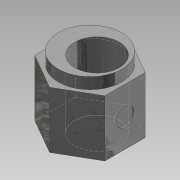
# Autodesk Inventor part: Eccentric M5 Spacer
Saved by Autodesk Inventor 2016 (Build 200138000, 138)
## iProperties
Created: 2013-06-19
Part Number: Eccentric M5 Spacer
Material: Stainless Steel
Document SubType Name: Modeling
Designer: Jon Hollander
Density: 8.08 g/cm^3
Mass: 1.9468 g
Surface Area: 3.90129 cm^2
Volume: 0.240941 cm^3
Appearance: Semi-Polished
Author: Jon Hollander
Autodesk Inventor part; units mm, degrees
ref_plane "YZ Plane" through (0, 0, 0) normal (1, 0, 0) x (0, 1, 0)
ref_plane "XZ Plane" through (0, 0, 0) normal (0, 1, 0) x (-1, 0, 0)
ref_plane "XY Plane" through (0, 0, 0) normal (0, 0, 1) x (1, 0, 0)
sketch "Sketch1" plane through (0, 0, 0) normal (0, 0, 1) x (1, 0, 0)
  line L0 (3.935, -2.2719) -> (0, -4.5437)
  line L1 (0, -4.5437) -> (-3.935, -2.2719)
  line L2 (-3.935, -2.2719) -> (-3.935, 2.2719)
  line L3 (-3.935, 2.2719) -> (0, 4.5437)
  line L4 (0, 4.5437) -> (3.935, 2.2719)
  line L5 (3.935, 2.2719) -> (3.935, -2.2719)
  circle A0 centre (0.79, 0) radius 2.5
  point P0 (0, 0)
  point P1 (0, 0)
  dimension "d0" = 7.87
  dimension "d1" = 0.79
  dimension "d2" = 5
  constraints: 12 end point, 2 coincident, 1 centre point, 1 horizontal alignment, 1 vertical, 13 other
  measures "d0" distance between parallel lines of L1 L4
  measures "d1" distance of point (0.79, 0) point (0, 0)
  measures "d2" diameter of A0
extrude "Extrusion1" add sketch "Sketch1" along normal blind 6.35
sketch "Sketch2" plane through (0, 0, 6.35) normal (0, 0, 1) x (1, 0, 0)
  circle A0 centre (0.79, 0) radius 2.5 projected
  circle A1 centre (0, 0) radius 3.555
  dimension "d5" = 7.11
  constraints: 1 centre point, 1 coincident
  measures "d5" diameter of A1
extrude "Extrusion2" add sketch "Sketch2" along normal blind 1.27
sketch "Sketch3" plane through (3.935, -2.2719, 0) normal (1, 0, 0) x (0, 0, -1)
  circle A0 centre (-3.175, 2.2719) radius 1
  point P0 (0, 2.2719)
  dimension "d8" = 2
  constraints: 1 centre point
  measures "d8" diameter of A0
extrude "Extrusion3" cut sketch "Sketch3" against normal blind 0.15
body "Solid1"
